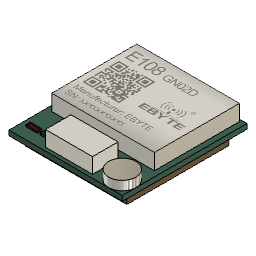
meshjoy-v02-case-fusion-v20 (Autodesk Fusion 360 archive; units mm, degrees)
design "E108-GN02D GPS Ebyte"
Autodesk Fusion 360 part; units mm, degrees
box "BoxPrimitive1" add length 22 width 20 height 0.9 placed x (0, 1, 0) y (-1, 0, 0) z (0, 0, 1) at (20, 0, 0) makes body 1
move_body "Align1" bodies 1 to x (1, 0, 0) y (0, 1, 0) z (0, 0, 1) at (-10, -11, -0.9)
sketch "Sketch2" plane through (0, 0, 0) normal (0, 0, 1) x (-1, 0, 0)
  line L0 (-10, -11) -> (10, -11)
  line L1 (10, -11) -> (10, 11)
  line L2 (10, 11) -> (-10, 11)
  line L3 (-10, 11) -> (-10, -11)
  line L4 (9.05, -10.6) -> (-9.05, -10.6)
  line L5 (-9.05, -10.6) -> (-9.05, 4.4)
  line L6 (-9.05, 4.4) -> (9.05, 4.4)
  line L7 (9.05, 4.4) -> (9.05, -10.6)
  line L8 (0, -11) -> (0, 11)
  line L9 (4.15, 5.9) -> (-4.15, 5.9)
  line L10 (-4.15, 5.9) -> (-4.15, 10.4)
  line L11 (-4.15, 10.4) -> (4.15, 10.4)
  line L12 (4.15, 10.4) -> (4.15, 5.9)
  circle A0 centre (-7.6, 8.6) radius 2.4
  line L13 (9, 8.2) -> (7, 8.2)
  line L14 (7, 8.2) -> (7, 9)
  line L15 (7, 9) -> (9, 9)
  line L16 (9, 9) -> (9, 8.2)
  line L17 (6.5, 8.2) -> (4.5, 8.2)
  line L18 (4.5, 8.2) -> (4.5, 9)
  line L19 (4.5, 9) -> (6.5, 9)
  line L20 (6.5, 9) -> (6.5, 8.2)
  point P0 (0, -10.6)
  point P1 (0, 10.4)
  dimension "d8" = 18.1
  dimension "d9" = 15
  dimension "d10" = 0.4
  dimension "d24" = 8.3
  dimension "d25" = 4.5
  dimension "d26" = 0.6
  dimension "d29" = 4.8
  dimension "d32" = 2
  dimension "d33" = 0.8
  dimension "d34" = 2
  dimension "d35" = 1
  dimension "d36" = 2
  dimension "d37" = 0.8
  dimension "d38" = 0.5
  dimension "d39" = 2
  constraint horizontal L4
  constraint vertical L5
  constraint horizontal L6
  constraint vertical L7
  constraint midpoint L0 L8.start
  constraint midpoint L2 L8.end
  constraint midpoint L4 P0
  constraint coincident L8 P0
  constraint horizontal L9
  constraint vertical L10
  constraint horizontal L11
  constraint vertical L12
  constraint midpoint L11 P1
  constraint coincident L8 P1
  constraint tangent L2 A0
  constraint tangent L3 A0
  constraint horizontal L13
  constraint vertical L14
  constraint horizontal L15
  constraint vertical L16
  constraint horizontal L17
  constraint vertical L18
  constraint horizontal L19
  constraint vertical L20
  measures "d8" distance of L4.start L4.end
  measures "d9" distance of L4.start L6.end
  measures "d10" distance of L0 L4
  measures "d24" distance of L9.start L9.end
  measures "d25" distance of L9.start L11.end
  measures "d26" distance of L2 L11
  measures "d29" diameter of A0
  measures "d32" distance of L13.start L13.end
  measures "d33" distance of L13.start L15.end
  measures "d34" distance of L2 L15
  measures "d35" distance of L1 L16
  measures "d36" distance of L17.start L17.end
  measures "d37" distance of L17.start L19.end
  measures "d38" distance of L14 L20
  measures "d39" distance of L2 L19
extrude "Extrude1" add sketch "Sketch2" along normal blind 2.8 separate body contours L4 L6 L7 L8 | L4 L5 L6 L8 makes body 2
sketch "Sketch3" plane through (0, 0, -0.9) normal (0, 0, -1) x (1, 0, 0)
  line L0 (-10, -11) -> (10, -11)
  line L1 (10, -11) -> (10, 11)
  line L2 (10, 11) -> (-10, 11)
  line L3 (-10, 11) -> (-10, -11)
  line L4 (8.7, -9.1) -> (-9.3, -9.1)
  line L5 (-9.3, -9.1) -> (-9.3, 8.9)
  line L6 (-9.3, 8.9) -> (8.7, 8.9)
  line L7 (8.7, 8.9) -> (8.7, -9.1)
  circle A0 centre (-1, 2.9) radius 1.5
  dimension "d13" = 18
  dimension "d14" = 18
  dimension "d15" = 1.9
  dimension "d16" = 0.7
  dimension "d17" = 3
  dimension "d18" = 9
  dimension "d19" = 12
  constraint horizontal L4
  constraint vertical L5
  constraint horizontal L6
  constraint vertical L7
  measures "d13" distance of L4.start L4.end
  measures "d14" distance of L4.start L6.end
  measures "d15" distance of L0 L4
  measures "d16" distance of L3 L5
  measures "d17" diameter of A0
  measures "d18" distance of L3 A0.centre
  measures "d19" distance of L4 A0.centre
extrude "Extrude2" add sketch "Sketch3" along normal blind 2.2 separate body contours L4 L5 L6 L7 | A0 makes body 3
extrude "Extrude3" add sketch "Sketch3" along normal up to surface (2.3 mm away) separate body contours A0 makes body 4
extrude "Extrude4" add sketch "Sketch2" along normal blind 2.7 separate body contours L8 L9 L10 L11 | L8 L9 L11 L12 makes body 5
extrude "Extrude5" add sketch "Sketch2" along normal blind 1.6 separate body contours A0 makes body 6
extrude "Extrude6" add sketch "Sketch2" along normal blind 0.3 separate body contours L13 L14 L15 L16 makes body 7
extrude "Extrude7" add sketch "Sketch2" along normal blind 0.3 separate body contours L17 L18 L19 L20 makes body 8
equation "d39 = d34"
named bodies: "PCB", "shield", "antenna", "connector", "battery", "LED red", "LED blue", "antenna tip"
